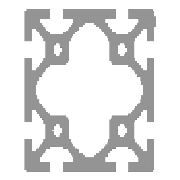
# Autodesk Inventor part: Item60x60
Saved by Autodesk Inventor 2024 (Build 280153020, 153B)
## iProperties
Created: 2023-08-07
Part Number: Item60x60
Material: Generisch
Description: Item60x60
Document SubType Name: Modeling
Designer: hol
Manufacturer: ITEM
Standards Organization: ISO
Language: de-DE
Size Designation: Item60x60
Categories: <MemberInstance><Categories><Category DisplayName="Profile" InternalName="089c4875-fa83-4c05-b084-43b9cc11f5ed" Mnemonic="GRDR"><CategoryParameter DisplayName="Masse pro Längeneinheit" InternalName="0bb95a10-148f-4027-a459-38d7b056702a" Mnemonic="shpmass"/><CategoryParameter DisplayName="Querschnittsfläche" InternalName="1ff91680-64b0-4202-b9a3-7fd3f94bba3b" Mnemonic="secarea"/><CategoryParameter DisplayName="Trägheitsradius (x)" InternalName="25778675-03e9-40c1-b6a8-4a9ed693320d" Mnemonic="gyrradx"/><CategoryParameter DisplayName="Torsion-Festigkeitsmodul" InternalName="26c1ec35-5026-4c63-ad0a-751cf684a536" Mnemonic="torrigmod"/><CategoryParameter DisplayName="Abstand zum Schwerpunkt X-X" InternalName="26c9bdb8-9c79-4b4f-a92e-8e197583c9c4" Mnemonic="grcendistX"/><CategoryParameter DisplayName="Alte Varianten-ID" InternalName="340afe4f-75d7-48d3-ab7d-943f3c3da468" Mnemonic="LegacyMemberID"/><CategoryParameter DisplayName="Basislänge" InternalName="42e34263-8f20-4d0e-ad48-bf1385b87c24" Mnemonic="shplen"/><CategoryParameter DisplayName="Trägheitsmoment (y)" InternalName="4b9f58ea-bced-460e-81ea-3d29ca5a49e3" Mnemonic="inermomy"/><CategoryParameter DisplayName="Trägheitsmoment (x)" InternalName="4cd780bc-73d7-43ac-917a-579e5cbd684d" Mnemonic="inermomx"/><CategoryParameter DisplayName="Benutzerdefinierter Basispunkt" InternalName="4f1d1b73-316d-484b-a3df-9cbabb16eb77" Mnemonic="shpBasePoint"/><CategoryParameter DisplayName="Objekthöhe" InternalName="50274e7d-5ac0-4796-92cb-c59e54983c67" Mnemonic="shpheig"/><CategoryParameter DisplayName="Widerstandsmoment (y)" InternalName="59eaa5e9-d227-48dc-b6c1-6920f96e0f95" Mnemonic="secmody"/><CategoryParameter DisplayName="Schnittbezeichnung" InternalName="5a64d034-428d-49c8-ba32-7619764de20f" Mnemonic="shpdes"/><CategoryParameter DisplayName="Widerstandsmoment (x)" InternalName="72cfad18-cf51-4ed4-aaa7-c6b224f8419f" Mnemonic="secmodx"/><CategoryParameter DisplayName="Drehrissmodul" InternalName="7c55a8dc-8844-49f9-a867-cc677b30ec9a" Mnemonic="torsecmod"/><CategoryParameter DisplayName="Objektbreite" InternalName="7c717d54-a18f-4666-b4d4-573cce22c62c" Mnemonic="shpwdth"/><CategoryParameter DisplayName="Zweite Objektdicke" InternalName="9251a8e1-85fd-4e47-af99-afdb762317d9" Mnemonic="shpthick2"/><CategoryParameter DisplayName="GG Erstellt" InternalName="9c666724-f362-4ea7-ac62-f6a007de5c69" Mnemonic="shpFGAuto"/><CategoryParameter DisplayName="Abstand zum Schwerpunkt Y-Y" InternalName="bcc4fb17-7af4-436a-8f8c-d0aa3b0248c5" Mnemonic="grcendistY"/><CategoryParameter DisplayName="Trägheitsradius (y)" InternalName="bfa18ebe-1636-4dbe-8d42-b263e0b73184" Mnemonic="gyrrady"/><CategoryParameter DisplayName="Objektdicke" InternalName="d109cf76-8eb4-42fc-9800-4409734adc67" Mnemonic="shpthick"/><CategoryParameter DisplayName="Koeffizient für Schubverschiebung" InternalName="de4c90c6-aaa8-468f-a335-6737b311b5d3" Mnemonic="shdispc"/><Category DisplayName="Sonstiges" InternalName="f02205ff-2390-476f-921c-0b3185f88e84" Mnemonic="OTHSHP"><CategoryParameter DisplayName="Trägheitsmoment (y)" InternalName="044c654e-f649-48ac-84cc-650a29ae31ca" Mnemonic="inermomy"/><CategoryParameter DisplayName="Objektdicke" InternalName="12b1a788-9233-48fd-a933-2df8ff42b15f" Mnemonic="shpthick"/><CategoryParameter DisplayName="Masse pro Längeneinheit" InternalName="2fd289d6-9394-4d2d-97e6-6659d7d4551d" Mnemonic="shpmass"/><CategoryParameter DisplayName="Trägheitsradius (y)" InternalName="743e1dfe-1bba-408b-b985-cf752b207386" Mnemonic="gyrrady"/><CategoryParameter DisplayName="Widerstandsmoment (y)" InternalName="88b8bff9-a616-4028-93d5-ed4f79680d13" Mnemonic="secmody"/><CategoryParameter DisplayName="Querschnittsfläche" InternalName="c46ecdf8-b6eb-4db9-8b25-30258930c1e3" Mnemonic="secarea"/><CategoryParameter DisplayName="Widerstandsmoment (x)" InternalName="cac70804-9d39-43bb-be17-56ea1f39a6c2" Mnemonic="secmodx"/><CategoryParameter DisplayName="Trägheitsmoment (x)" InternalName="ec6737bc-264f-43ed-b0bd-f6d410c2718d" Mnemonic="inermomx"/><CategoryParameter DisplayName="Trägheitsradius (x)" InternalName="ee72c61e-565e-4fd6-b448-66e1e1abcb7e" Mnemonic="gyrradx"/></Category></Category><Category DisplayName="Datentyp" InternalName="23b78d0f-2648-40c6-8793-ca6db495c9e8" Mnemonic="DATATYPE"><CategoryParameter DisplayName="Anzeigename" InternalName="05415f3d-3907-474b-a020-eb9d644f4cf3" Mnemonic="DISPLAYNAME"/><CategoryParameter DisplayName="Norm" InternalName="0c0a119c-1e12-4c84-803f-101930972f5e" Mnemonic="STANDARD"/><CategoryParameter DisplayName="Beschreibung" InternalName="13903e3d-64b1-4950-80da-f627842ea37f" Mnemonic="DESCRIPTION"/><CategoryParameter DisplayName="Bezeichnung" InternalName="2675968c-4ce5-49e0-a4f5-552d29089031" Mnemonic="DESIGNATION"/><CategoryParameter DisplayName="Standardzeile" InternalName="2af9ec52-faaa-4026-b378-f9fa4afca842" Mnemonic="DEFAULTROW"/><CategoryParameter DisplayName="Ordnername" InternalName="3f06958e-8713-4116-9be7-ed6184ecc97b" Mnemonic="FOLDERNAME"/><CategoryParameter DisplayName="Revisionsanleitung" InternalName="45a75005-10b1-4dfc-8d6d-dfe629f0b93c" Mnemonic="REVISIONGUID"/><CategoryParameter DisplayName="Dateiname" InternalName="8b46a4cc-9585-4fed-90c3-899f57e09a73" Mnemonic="FILENAME"/><CategoryParameter DisplayName="Normungsorganisation" InternalName="8f5914e1-4693-403f-8ab5-d37768198c9d" Mnemonic="STDSORG"/><CategoryParameter DisplayName="Gruppenversion" InternalName="914462f6-6e19-4b14-ba84-155b9680b1d0" Mnemonic="FAMILYREVISION"/><CategoryParameter DisplayName="Normrevision" InternalName="91d5a463-65c2-4fde-b823-3b7fea5e8e17" Mnemonic="STANDARDREVISION"/><CategoryParameter DisplayName="Variantenrevision" InternalName="a65d44b9-392f-4f4f-857b-e4b3d54996fe" Mnemonic="MEMBERREVISION"/><CategoryParameter DisplayName="ClipFormat" InternalName="bc51e27b-3422-4e78-93ef-cec197ddf230" Mnemonic="CLIPFORMAT"/><CategoryParameter DisplayName="Hersteller" InternalName="cd6c7a72-a28a-4e50-99a9-2c7f4e13e5ad" Mnemonic="MANUFACTURER"/><CategoryParameter DisplayName="InternerName" InternalName="cf1d0246-76d9-4b4a-8305-fa0409afb5c1" Mnemonic="INTERNALNAME"/><CategoryParameter DisplayName="IstMetrisch" InternalName="e2385c5b-1ea4-4823-96a8-8de651266ec3" Mnemonic="ISMETRIC"/><Category DisplayName="Bauteil" InternalName="c0e0b642-3bcb-4cc8-9e80-f96d35c4afa4" Mnemonic="PART"><CategoryParameter DisplayName="Bauteilnummer" InternalName="016b6077-bfbe-49bd-92c9-d8d59c39c941" Mnemonic="PARTNUMBER"/><CategoryParameter DisplayName="Bestandsnummer" InternalName="4dba7c1c-e26c-444e-836c-b08b433409a8" Mnemonic="STOCKNUMBER"/><CategoryParameter DisplayName="Materialschlüssel" InternalName="5c9a8adb-dd2b-4535-b97f-0a94a95fe41f" Mnemonic="MATERIALKEY"/><CategoryParameter DisplayName="Material" InternalName="818a152a-d3c3-49ca-80ee-df7d91421b8e" Mnemonic="MATERIAL"/></Category></Category></Categories><FamilyTemplate Id="Item60x60"><FamilyTemplateParameters><FamilyTemplateParameter ObjectType="kModelParameterObject" ValueType="xs:double" Id="12" ObjectReferenceKey="d0"/><FamilyTemplateParameter ObjectType="kPartComponentDefinitionObject" ValueType="xs:string" Id="23" SubObjectId="Material"/><FamilyTemplateParameter ObjectType="kPropertyObject" ValueType="xs:string" Id="26" ObjectReferenceKey="{32853F0F-3444-11d1-9E93-0060B03C1CA6}" SubObjectId="5"/><FamilyTemplateParameter ObjectType="kPropertyObject" ValueType="xs:string" Id="27" ObjectReferenceKey="{32853F0F-3444-11d1-9E93-0060B03C1CA6}" SubObjectId="52"/></FamilyTemplateParameters></FamilyTemplate><CategoryParameterMap><ParamToTemplateMap><ParamToTemplate CategoryParameter="//CategoryParameter[@InternalName='cf1d0246-76d9-4b4a-8305-fa0409afb5c1']" ConstantValue="55f69150-1e01-4d98-b6af-d06e6a2b300a"/><ParamToTemplate CategoryParameter="//CategoryParameter[@InternalName='45a75005-10b1-4dfc-8d6d-dfe629f0b93c']" ConstantValue="875fef43-ba4c-4005-943e-916aab125456"/><ParamToTemplate CategoryParameter="//CategoryParameter[@InternalName='3f06958e-8713-4116-9be7-ed6184ecc97b']" ConstantValue="Item Profile"/><ParamToTemplate CategoryParameter="//CategoryParameter[@InternalName='8f5914e1-4693-403f-8ab5-d37768198c9d']" ConstantValue="ISO"/><ParamToTemplate CategoryParameter="//CategoryParameter[@InternalName='0c0a119c-1e12-4c84-803f-101930972f5e']" TemplateParameter="18"/><ParamToTemplate CategoryParameter="//CategoryParameter[@InternalName='91d5a463-65c2-4fde-b823-3b7fea5e8e17']" TemplateParameter="19"/><ParamToTemplate CategoryParameter="//CategoryParameter[@InternalName='cd6c7a72-a28a-4e50-99a9-2c7f4e13e5ad']" ConstantValue="ITEM"/><ParamToTemplate CategoryParameter="//CategoryParameter[@InternalName='13903e3d-64b1-4950-80da-f627842ea37f']" ConstantValue="Item60x60"/><ParamToTemplate CategoryParameter="//CategoryParameter[@InternalName='05415f3d-3907-474b-a020-eb9d644f4cf3']" ConstantValue="Item Profile"/><ParamToTemplate CategoryParameter="//CategoryParameter[@InternalName='914462f6-6e19-4b14-ba84-155b9680b1d0']" ConstantValue="11"/><ParamToTemplate CategoryParameter="//CategoryParameter[@InternalName='bc51e27b-3422-4e78-93ef-cec197ddf230']" ConstantValue="CF_INVENTOR.STDPARTS"/><ParamToTemplate CategoryParameter="//CategoryParameter[@InternalName='e2385c5b-1ea4-4823-96a8-8de651266ec3']" ConstantValue="true"/><ParamToTemplate CategoryParameter="//CategoryParameter[@InternalName='2af9ec52-faaa-4026-b378-f9fa4afca842']" ConstantValue="1"/><ParamToTemplate CategoryParameter="//CategoryParameter[@InternalName='9c666724-f362-4ea7-ac62-f6a007de5c69']" ConstantValue="1"/><ParamToTemplate CategoryParameter="//CategoryParameter[@InternalName='8b46a4cc-9585-4fed-90c3-899f57e09a73']" ConstantValue="Generisch-Item60x60-10"/><ParamToTemplate CategoryParameter="//CategoryParameter[@InternalName='a65d44b9-392f-4f4f-857b-e4b3d54996fe']" ConstantValue="fd1726a2-92ec-4608-a585-b6133f5c2eec"/><ParamToTemplate CategoryParameter="//CategoryParameter[@InternalName='a65d44b9-392f-4f4f-857b-e4b3d54996fe']" ConstantValue="fd1726a2-92ec-4608-a585-b6133f5c2eec"/><ParamToTemplate CategoryParameter="//CategoryParameter[@InternalName='2675968c-4ce5-49e0-a4f5-552d29089031']" TemplateParameter="27"/><ParamToTemplate CategoryParameter="//CategoryParameter[@InternalName='818a152a-d3c3-49ca-80ee-df7d91421b8e']" TemplateParameter="23"/><ParamToTemplate CategoryParameter="//CategoryParameter[@InternalName='016b6077-bfbe-49bd-92c9-d8d59c39c941']" TemplateParameter="26"/><ParamToTemplate CategoryParameter="//CategoryParameter[@InternalName='42e34263-8f20-4d0e-ad48-bf1385b87c24']" TemplateParameter="12"/></ParamToTemplateMap></CategoryParameterMap></MemberInstance>
Density: 1 g/cm^3
Appearance: Vorgabe
IsCustomPart: 1
_CCFamilyDisplayName: Item Profile - Item60x60
_FrameMemberDoc: Frame Member File
_Version: 25.0.0
_GetPNFromCC: 1
Author: hol
G_L: 1000,000 mm
G_W: 60,000 mm
G_H: 60,000 mm
Autodesk Inventor part; units mm, degrees
ref_plane "XZ Plane" through (0, 0, 0) normal (0, 1, 0) x (-1, 0, 0)
ref_plane "Startebene" through (0, 0, 0) normal (1, 0, 0) x (0, 1, 0)
ref_plane "Endebene" through (1000, 0, 0) normal (1, 0, 0) x (0, 1, 0)
sketch "Skizze" plane through (0, 0, 0) normal (1, 0, 0) x (0, 1, 0)
  arc A0 (25.868, 56.4338) -> (26.668, 57.2338) centre (25.868, 57.2338) ccw
  line L0 (26.668, 57.2338) -> (26.668, 58.4338)
  arc A1 (26.668, 58.4338) -> (25.668, 59.4338) centre (25.668, 58.4338) ccw
  line L1 (25.668, 59.4338) -> (3.868, 59.4338)
  arc A2 (3.868, 59.4338) -> (2.868, 58.4338) centre (3.868, 58.4338) ccw
  line L2 (2.868, 58.4338) -> (2.868, 57.2338)
  arc A3 (2.868, 57.2338) -> (3.668, 56.4338) centre (3.668, 57.2338) ccw
  line L3 (3.668, 56.4338) -> (6.8956, 56.4338)
  arc A4 (7.6186, 54.6885) -> (6.8956, 56.4338) centre (6.8956, 55.4114) ccw
  line L4 (7.6186, 54.6885) -> (3.4925, 50.5624)
  arc A5 (1.3712, 49.6838) -> (3.4925, 50.5624) centre (1.3712, 52.6838) ccw
  line L5 (1.3712, 49.6838) -> (-1.8352, 49.6838)
  arc A6 (-3.9565, 50.5624) -> (-1.8352, 49.6838) centre (-1.8352, 52.6838) ccw
  line L6 (-3.9565, 50.5624) -> (-8.0826, 54.6885)
  arc A7 (-7.3596, 56.4338) -> (-8.0826, 54.6885) centre (-7.3596, 55.4114) ccw
  line L7 (-7.3596, 56.4338) -> (-4.132, 56.4338)
  arc A8 (-4.132, 56.4338) -> (-3.332, 57.2338) centre (-4.132, 57.2338) ccw
  line L8 (-3.332, 57.2338) -> (-3.332, 58.4338)
  arc A9 (-3.332, 58.4338) -> (-4.332, 59.4338) centre (-4.332, 58.4338) ccw
  line L9 (-4.332, 59.4338) -> (-12.232, 59.4338)
  arc A10 (-12.232, 59.4338) -> (-15.232, 56.4338) centre (-12.232, 56.4338) ccw
  line L10 (-15.232, 56.4338) -> (-15.232, 48.5338)
  arc A11 (-15.232, 48.5338) -> (-14.232, 47.5338) centre (-14.232, 48.5338) ccw
  line L11 (-14.232, 47.5338) -> (-13.032, 47.5338)
  arc A12 (-13.032, 47.5338) -> (-12.232, 48.3338) centre (-13.032, 48.3338) ccw
  line L12 (-12.232, 48.3338) -> (-12.232, 51.5614)
  arc A13 (-10.4867, 52.2843) -> (-12.232, 51.5614) centre (-11.2096, 51.5614) ccw
  line L13 (-10.4867, 52.2843) -> (-6.3607, 48.1583)
  arc A14 (-5.482, 46.037) -> (-6.3607, 48.1583) centre (-8.482, 46.037) ccw
  line L14 (-5.482, 46.037) -> (-5.482, 42.8306)
  arc A15 (-6.3607, 40.7092) -> (-5.482, 42.8306) centre (-8.482, 42.8306) ccw
  line L15 (-6.3607, 40.7092) -> (-10.4867, 36.5832)
  arc A16 (-12.232, 37.3061) -> (-10.4867, 36.5832) centre (-11.2096, 37.3061) ccw
  line L16 (-12.232, 37.3061) -> (-12.232, 40.5338)
  arc A17 (-12.232, 40.5338) -> (-13.032, 41.3338) centre (-13.032, 40.5338) ccw
  line L17 (-13.032, 41.3338) -> (-14.232, 41.3338)
  arc A18 (-14.232, 41.3338) -> (-15.232, 40.3338) centre (-14.232, 40.3338) ccw
  line L18 (-15.232, 40.3338) -> (-15.232, 18.5338)
  arc A19 (-15.232, 18.5338) -> (-14.232, 17.5338) centre (-14.232, 18.5338) ccw
  line L19 (-14.232, 17.5338) -> (-13.032, 17.5338)
  arc A20 (-13.032, 17.5338) -> (-12.232, 18.3338) centre (-13.032, 18.3338) ccw
  line L20 (-12.232, 18.3338) -> (-12.232, 21.5614)
  arc A21 (-10.4867, 22.2843) -> (-12.232, 21.5614) centre (-11.2096, 21.5614) ccw
  line L21 (-10.4867, 22.2843) -> (-6.3607, 18.1583)
  arc A22 (-5.482, 16.037) -> (-6.3607, 18.1583) centre (-8.482, 16.037) ccw
  line L22 (-5.482, 16.037) -> (-5.482, 12.8306)
  arc A23 (-6.3607, 10.7092) -> (-5.482, 12.8306) centre (-8.482, 12.8306) ccw
  line L23 (-6.3607, 10.7092) -> (-10.4867, 6.5832)
  arc A24 (-12.232, 7.3061) -> (-10.4867, 6.5832) centre (-11.2096, 7.3061) ccw
  line L24 (-12.232, 7.3061) -> (-12.232, 10.5338)
  arc A25 (-12.232, 10.5338) -> (-13.032, 11.3338) centre (-13.032, 10.5338) ccw
  line L25 (-13.032, 11.3338) -> (-14.232, 11.3338)
  arc A26 (-14.232, 11.3338) -> (-15.232, 10.3338) centre (-14.232, 10.3338) ccw
  line L26 (-15.232, 10.3338) -> (-15.232, 2.4338)
  arc A27 (-15.232, 2.4338) -> (-12.232, -0.5662) centre (-12.232, 2.4338) ccw
  line L27 (-12.232, -0.5662) -> (-4.332, -0.5662)
  arc A28 (-4.332, -0.5662) -> (-3.332, 0.4338) centre (-4.332, 0.4338) ccw
  line L28 (-3.332, 0.4338) -> (-3.332, 1.6338)
  arc A29 (-3.332, 1.6338) -> (-4.132, 2.4338) centre (-4.132, 1.6338) ccw
  line L29 (-4.132, 2.4338) -> (-7.3596, 2.4338)
  arc A30 (-8.0826, 4.179) -> (-7.3596, 2.4338) centre (-7.3596, 3.4561) ccw
  line L30 (-8.0826, 4.179) -> (-3.9565, 8.3051)
  arc A31 (-1.8352, 9.1838) -> (-3.9565, 8.3051) centre (-1.8352, 6.1838) ccw
  line L31 (-1.8352, 9.1838) -> (1.3712, 9.1838)
  arc A32 (3.4925, 8.3051) -> (1.3712, 9.1838) centre (1.3712, 6.1838) ccw
  line L32 (3.4925, 8.3051) -> (7.6186, 4.179)
  arc A33 (6.8956, 2.4338) -> (7.6186, 4.179) centre (6.8956, 3.4561) ccw
  line L33 (6.8956, 2.4338) -> (3.668, 2.4338)
  arc A34 (3.668, 2.4338) -> (2.868, 1.6338) centre (3.668, 1.6338) ccw
  line L34 (2.868, 1.6338) -> (2.868, 0.4338)
  arc A35 (2.868, 0.4338) -> (3.868, -0.5662) centre (3.868, 0.4338) ccw
  line L35 (3.868, -0.5662) -> (25.668, -0.5662)
  arc A36 (25.668, -0.5662) -> (26.668, 0.4338) centre (25.668, 0.4338) ccw
  line L36 (26.668, 0.4338) -> (26.668, 1.6338)
  arc A37 (26.668, 1.6338) -> (25.868, 2.4338) centre (25.868, 1.6338) ccw
  line L37 (25.868, 2.4338) -> (22.6404, 2.4338)
  arc A38 (21.9174, 4.179) -> (22.6404, 2.4338) centre (22.6404, 3.4561) ccw
  line L38 (21.9174, 4.179) -> (26.0435, 8.3051)
  arc A39 (28.1648, 9.1838) -> (26.0435, 8.3051) centre (28.1648, 6.1838) ccw
  line L39 (28.1648, 9.1838) -> (31.3712, 9.1838)
  arc A40 (33.4925, 8.3051) -> (31.3712, 9.1838) centre (31.3712, 6.1838) ccw
  line L40 (33.4925, 8.3051) -> (37.6186, 4.179)
  arc A41 (36.8956, 2.4338) -> (37.6186, 4.179) centre (36.8956, 3.4561) ccw
  line L41 (36.8956, 2.4338) -> (33.668, 2.4338)
  arc A42 (33.668, 2.4338) -> (32.868, 1.6338) centre (33.668, 1.6338) ccw
  line L42 (32.868, 1.6338) -> (32.868, 0.4338)
  arc A43 (32.868, 0.4338) -> (33.868, -0.5662) centre (33.868, 0.4338) ccw
  line L43 (33.868, -0.5662) -> (41.768, -0.5662)
  arc A44 (41.768, -0.5662) -> (44.768, 2.4338) centre (41.768, 2.4338) ccw
  line L44 (44.768, 2.4338) -> (44.768, 10.3338)
  arc A45 (44.768, 10.3338) -> (43.768, 11.3338) centre (43.768, 10.3338) ccw
  line L45 (43.768, 11.3338) -> (42.568, 11.3338)
  arc A46 (42.568, 11.3338) -> (41.768, 10.5338) centre (42.568, 10.5338) ccw
  line L46 (41.768, 10.5338) -> (41.768, 7.3061)
  arc A47 (40.0227, 6.5832) -> (41.768, 7.3061) centre (40.7456, 7.3061) ccw
  line L47 (40.0227, 6.5832) -> (35.8967, 10.7092)
  arc A48 (35.018, 12.8306) -> (35.8967, 10.7092) centre (38.018, 12.8306) ccw
  line L48 (35.018, 12.8306) -> (35.018, 16.037)
  arc A49 (35.8967, 18.1583) -> (35.018, 16.037) centre (38.018, 16.037) ccw
  line L49 (35.8967, 18.1583) -> (40.0227, 22.2843)
  arc A50 (41.768, 21.5614) -> (40.0227, 22.2843) centre (40.7456, 21.5614) ccw
  line L50 (41.768, 21.5614) -> (41.768, 18.3338)
  arc A51 (41.768, 18.3338) -> (42.568, 17.5338) centre (42.568, 18.3338) ccw
  line L51 (42.568, 17.5338) -> (43.768, 17.5338)
  arc A52 (43.768, 17.5338) -> (44.768, 18.5338) centre (43.768, 18.5338) ccw
  line L52 (44.768, 18.5338) -> (44.768, 40.3338)
  arc A53 (44.768, 40.3338) -> (43.768, 41.3338) centre (43.768, 40.3338) ccw
  line L53 (43.768, 41.3338) -> (42.568, 41.3338)
  arc A54 (42.568, 41.3338) -> (41.768, 40.5338) centre (42.568, 40.5338) ccw
  line L54 (41.768, 40.5338) -> (41.768, 37.3061)
  arc A55 (40.0227, 36.5832) -> (41.768, 37.3061) centre (40.7456, 37.3061) ccw
  line L55 (40.0227, 36.5832) -> (35.8967, 40.7092)
  arc A56 (35.018, 42.8306) -> (35.8967, 40.7092) centre (38.018, 42.8306) ccw
  line L56 (35.018, 42.8306) -> (35.018, 46.037)
  arc A57 (35.8967, 48.1583) -> (35.018, 46.037) centre (38.018, 46.037) ccw
  line L57 (35.8967, 48.1583) -> (40.0227, 52.2843)
  arc A58 (41.768, 51.5614) -> (40.0227, 52.2843) centre (40.7456, 51.5614) ccw
  line L58 (41.768, 51.5614) -> (41.768, 48.3338)
  arc A59 (41.768, 48.3338) -> (42.568, 47.5338) centre (42.568, 48.3338) ccw
  line L59 (42.568, 47.5338) -> (43.768, 47.5338)
  arc A60 (43.768, 47.5338) -> (44.768, 48.5338) centre (43.768, 48.5338) ccw
  line L60 (44.768, 48.5338) -> (44.768, 56.4338)
  arc A61 (44.768, 56.4338) -> (41.768, 59.4338) centre (41.768, 56.4338) ccw
  line L61 (41.768, 59.4338) -> (33.868, 59.4338)
  arc A62 (33.868, 59.4338) -> (32.868, 58.4338) centre (33.868, 58.4338) ccw
  line L62 (32.868, 58.4338) -> (32.868, 57.2338)
  arc A63 (32.868, 57.2338) -> (33.668, 56.4338) centre (33.668, 57.2338) ccw
  line L63 (33.668, 56.4338) -> (36.8956, 56.4338)
  arc A64 (37.6186, 54.6885) -> (36.8956, 56.4338) centre (36.8956, 55.4114) ccw
  line L64 (37.6186, 54.6885) -> (33.4925, 50.5624)
  arc A65 (31.3712, 49.6838) -> (33.4925, 50.5624) centre (31.3712, 52.6838) ccw
  line L65 (31.3712, 49.6838) -> (28.1648, 49.6838)
  arc A66 (26.0435, 50.5624) -> (28.1648, 49.6838) centre (28.1648, 52.6838) ccw
  line L66 (26.0435, 50.5624) -> (21.9174, 54.6885)
  arc A67 (22.6404, 56.4338) -> (21.9174, 54.6885) centre (22.6404, 55.4114) ccw
  line L67 (22.6404, 56.4338) -> (25.868, 56.4338)
  line L68 (-3.9565, 20.5624) -> (-8.5852, 25.1911)
  arc A68 (-8.5852, 33.6764) -> (-8.5852, 25.1911) centre (-4.3426, 29.4338) ccw
  line L69 (-8.5852, 33.6764) -> (-3.9565, 38.3051)
  arc A69 (-1.8352, 39.1838) -> (-3.9565, 38.3051) centre (-1.8352, 36.1838) ccw
  line L70 (-1.8352, 39.1838) -> (3.0977, 39.1838)
  arc A70 (3.0977, 39.1838) -> (3.4512, 39.3302) centre (3.0977, 39.6838) ccw
  line L71 (3.4512, 39.3302) -> (4.8715, 40.7505)
  arc A71 (4.8715, 40.7505) -> (5.018, 41.1041) centre (4.518, 41.1041) ccw
  line L72 (5.018, 41.1041) -> (5.018, 46.037)
  arc A72 (5.8967, 48.1583) -> (5.018, 46.037) centre (8.018, 46.037) ccw
  line L73 (5.8967, 48.1583) -> (10.5254, 52.787)
  arc A73 (19.0106, 52.787) -> (10.5254, 52.787) centre (14.768, 48.5443) ccw
  line L74 (19.0106, 52.787) -> (23.6393, 48.1583)
  arc A74 (24.518, 46.037) -> (23.6393, 48.1583) centre (21.518, 46.037) ccw
  line L75 (24.518, 46.037) -> (24.518, 41.1041)
  arc A75 (24.518, 41.1041) -> (24.6644, 40.7505) centre (25.018, 41.1041) ccw
  line L76 (24.6644, 40.7505) -> (26.0848, 39.3302)
  arc A76 (26.0848, 39.3302) -> (26.4383, 39.1838) centre (26.4383, 39.6838) ccw
  line L77 (26.4383, 39.1838) -> (31.3712, 39.1838)
  arc A77 (33.4925, 38.3051) -> (31.3712, 39.1838) centre (31.3712, 36.1838) ccw
  line L78 (33.4925, 38.3051) -> (38.1212, 33.6764)
  arc A78 (38.1212, 25.1911) -> (38.1212, 33.6764) centre (33.8785, 29.4338) ccw
  line L79 (38.1212, 25.1911) -> (33.4925, 20.5624)
  arc A79 (31.3712, 19.6838) -> (33.4925, 20.5624) centre (31.3712, 22.6838) ccw
  line L80 (31.3712, 19.6838) -> (26.4383, 19.6838)
  arc A80 (26.4383, 19.6838) -> (26.0848, 19.5373) centre (26.4383, 19.1838) ccw
  line L81 (26.0848, 19.5373) -> (24.6644, 18.117)
  arc A81 (24.6644, 18.117) -> (24.518, 17.7634) centre (25.018, 17.7634) ccw
  line L82 (24.518, 17.7634) -> (24.518, 12.8306)
  arc A82 (23.6393, 10.7092) -> (24.518, 12.8306) centre (21.518, 12.8306) ccw
  line L83 (23.6393, 10.7092) -> (19.0106, 6.0806)
  arc A83 (10.5254, 6.0806) -> (19.0106, 6.0806) centre (14.768, 10.3232) ccw
  line L84 (10.5254, 6.0806) -> (5.8967, 10.7092)
  arc A84 (5.018, 12.8306) -> (5.8967, 10.7092) centre (8.018, 12.8306) ccw
  line L85 (5.018, 12.8306) -> (5.018, 17.7634)
  arc A85 (5.018, 17.7634) -> (4.8715, 18.117) centre (4.518, 17.7634) ccw
  line L86 (4.8715, 18.117) -> (3.4512, 19.5373)
  arc A86 (3.4512, 19.5373) -> (3.0977, 19.6838) centre (3.0977, 19.1838) ccw
  line L87 (3.0977, 19.6838) -> (-1.8352, 19.6838)
  arc A87 (-3.9565, 20.5624) -> (-1.8352, 19.6838) centre (-1.8352, 22.6838) ccw
  circle A88 centre (-0.232, 14.4338) radius 2.5
  circle A89 centre (29.768, 14.4338) radius 2.5
  circle A90 centre (29.768, 44.4338) radius 2.5
  circle A91 centre (-0.232, 44.4338) radius 2.5
  point P0 (0, 0)
  point P1 (0, 0)
  constraints: 176 end point, 176 point on circle, 92 centre point, 1 coincident
extrude "Körper" add sketch "Skizze" along normal up to surface (1000 mm away) from surface at 0
sketch "Skizze8" plane through (0, 0, 0) normal (1, 0, 0) x (0, 1, 0)
  line L0 (0, 0) -> (10, 0)
ref_plane "Arbeitsebene6" through (0, 0, 0) normal (0, 0, -1) x (0, 1, 0)
sketch "Skizze9" plane through (0, 0, 0) normal (0, 0, -1) x (0, 1, 0)
  line L0 (-2, 0) -> (12, 0)
  line L1 (-2, 1000) -> (12, 1000)
  dimension "d7" = 1000
  measures "d7" distance between parallel lines of L0 L1
equation "\"G_OFFSET_START\" = 0"
equation "\"G_OFFSET_END\" = 0"
equation "\"G_L\" = d7"
